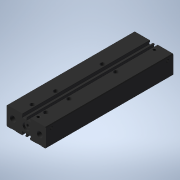
# Autodesk Inventor part: 529120 DFM---16-160-B-P-A-KF---(ZR) 150
Saved by Autodesk Inventor 2021 (Build 250183000, 183)
## iProperties
Created: 2025-06-19
Part Number: 529120 DFM---16-160-B-P-A-KF---(ZR) 150
Material: Generic
Catalog Web Link: www.cadenas.de
Description: DFM-B-(ZR)-Guide unit
Vendor: FESTO
Document SubType Name: Modeling
Designer: psAdmin
Manufacturer: FESTO
Mass: 360.15 g
Surface Area: 842.869 cm^2
Volume: 360.15 cm^3
Density: 1 g/cm^3
Appearance: PSOLRGB-175-175-175
Category: PARTsolutions
Company: FESTO
Title: 529120 DFM---16-160-B-P-A-KF---(ZR) 150
Author: Cadenas PARTsolutions
Comments: Guide unit
PSOL_IDENT_0: {$CADENAS_DATA/23d-libs/festo/parts/d/dfm/parts/dfm_b_z.prj},259 {VTYP=3D},{NB=529120 DFM---16-160-B
PSOL_IDENT_1: -P-A-KF---(ZR) 150},{LINA=529120 DFM---16-160-B-P-A-KF---(ZR) 150},{NN=DFM-B-(ZR)},{DATE=04.04.2025
PSOL_IDENT_2: 09:41:30},{GEOMDATE=04.04.2025 09:12:00},{VERSION=},{LINEID=550},{WBVAR=GEW,XHUB,CUSH,F,JUST},{WBNUM
PSOL_IDENT_3: ERIC=XHUB,CUSH,F,JUST}  {NB=529120 DFM---16-160-B-P-A-KF---(ZR) 150},{LINA=529120 DFM---16-160-B-P-A
PSOL_IDENT_4: -KF---(ZR) 150},{KT=1},{TNR=529120},{TYP=DFM},{GEW=-},{KDM=16},{D11=4.300},{XHUB=150},{HUB=160},{HUB
PSOL_IDENT_5: 1=[10:200]},{G=B},{CUSH=1},{F=2},{JUST=0},{VERS=1},{B1=67.000},{B2=65.000},{B3=45.000},{B4=4.500},{B
PSOL_IDENT_6: 5=58.000},{B6=22.000},{B7=23.000},{B8=23.500},{B9=20.000},{B10=10.500},{B11=46.000},{B12=9.500},{B13=
PSOL_IDENT_7: 46.000},{B14=21.300},{B15=24.400},{B16A=33.500},{B17A=0.000},{B18A=0.000},{B19A=0.000},{B20=0.000},{
PSOL_IDENT_8: B21=0.000},{D1=M 5},{D1P=5.000},{D1KDR=4.134},{D2=7.500},{D3=9.000},{D4=M 5},{D4P=5.000},{D4KDR=4.13
PSOL_IDENT_9: 4},{D5=5.000},{D6=4.3},{D6P=4.300},{D6KDR=3.242},{D7=10},{D7GF=12.000},{D7KF=10.000},{D8=5.000},{D9=
PSOL_IDENT_10: M 4},{D9P=4.000},{D9KDR=3.242},{D10=6.000},{FN=2},{FT=-KF},{E1=M 5},{EEMM=5.000},{EEKDR=4.134},{FE=
PSOL_IDENT_11: 0, '-', 1, 'AJ', 2, 'EJ', 3, 'AJ+EJ'},{H1=32.000},{H2=30.000},{H3=26.500},{H4=4.000},{H5=24.000},{H6=
PSOL_IDENT_12: 4.000},{H7=24.000},{H8=16.000},{H9=7.400},{H10=20.000},{H11=16.000},{H12A=16.000},{H13A=0.000},{H14A=
PSOL_IDENT_13: 16.000},{L1=264},{L2=58.000},{L3=10.000},{L4=12.000},{L5=9.800},{L6A=9.300},{L7=34},{L8=22.000},{L9=
PSOL_IDENT_14: 40},{L10=34.000},{L11=120},{L12=5.000},{L13A=4.000},{L14=0},{L15=0},{L16=0},{P1=0.000},{T1=12.000},{
PSOL_IDENT_15: T2=4.600},{T3=2.100},{T4=10.000},{T5=1.000},{T6=0.000},{T7=0.000},{T8=0.000},{T9=0.000},{SW1=10.000}
PSOL_IDENT_16: ,{SW2=10.000},{SW3=17.000},{SW4=0.000},{SW4D=0.000},{SW4KDR=0.000},{SW4M=0.000},{SW5=0.000},{SW6=0.0
PSOL_IDENT_17: 00},{SW7=0.000},{SW8=0.000},{SW9=0.000},{SW10=0.000},{SW2D=6.000},{SW2T=4.000},{ZZ=0},{MOD=1},{BR=0.
PSOL_IDENT_18: 000},{YB1=0.000},{YD1=0.000},{YD2=0.000},{YD3=0.000},{YD4=0.000},{YL1=0.000},{YL2=0.000},{YL3=0.000}
PSOL_IDENT_19: ,{YL4=0.000},{YL5=0.000},{YL6=0.000},{YL7=0.000},{YL14=0.000},{L14A=107.900},{L14Y=0.000},{L15A=0.00
PSOL_IDENT_20: 0},{L15Y=0.000},{L16A=107.900},{L16Y=0.000},{CUSHT=-P},{CUSHN=1},{JT=},{B16=0},{B17=0},{B18=0},{B19=
PSOL_IDENT_21: 0},{H12=0},{H13=0},{H14=0},{L6=0},{L13=0},{PPV1= 1, 'P', 2, 'PPV'},{PPV2= 1, 'P', 2, 'PPV'},{PPV= 1,
PSOL_IDENT_22: 'P', 2, 'PPV'},{JU= 0, '-', 1, 'AJ', 2, 'EJ', 3, 'AJ+EJ'},{FE1= 0, '-'},{VER=1.000},{RR=0.000},{VER
PSOL_IDENT_23: O=2},{A1=0.000},{A2=0.000},{A3=0.000},{A3D=0.000},{A4=0.000},{A5=0.000},{A6=0.000},{A7=0.000},{A8=0.
PSOL_IDENT_24: 000},{AD9=0.000},{A10=0.000},{A11=0.000},{A11D=0},{A12=0.000},{A13=0.000},{A14=0.000},{A15=0.000},{A
PSOL_IDENT_25: 16=0.000},{A17=0.000},{NPT=0},{BB=0.000},{LPPV=0.000},{DPPV=0.000},{LSLOT=8.000},{TSLOT=6.100},{YD33=
PSOL_IDENT_26: 0.000},{LD33=0.000}
NB: 529120 DFM---16-160-B-P-A-KF---(ZR) 150
NN: DFM-B-(ZR)
NT: Guide unit
NBSYN: $TNR. $TYP.-$GEW.-$KDM.-$HUB.-$G.$CUSHT.-A$FT.$JT.---(ZR) $XHUB.
LINA: 529120 DFM---16-160-B-P-A-KF---(ZR) 150
CATALOG: Festo
TNR: 529120
TYP: DFM
GEW: -
KDM: 16
D11: 4.3
XHUB: 150
HUB: 160
HUB1: [10:200]
G: B
CUSH: P
F: KF
JUST: -
B1: 67
B2: 65
B3: 45
B4: 4.5
B5: 58
B6: 22
B7: 23
B8: 23.5
B9: 20
B10: 10.5
B11: 46
B12: 9.5
B13: 46
B14: 21.3
B15: 24.4
B16A: 33.5
B17A: 0
B18A: 0
B19A: 0
B20: 0
B21: 0
D1: M 5
D1P: 5
D1KDR: 4.134
D2: 7.5
D3: 9
D4: M 5
D4P: 5
D4KDR: 4.134
D5: 5
D6: 4.3
D6P: 4.3
D6KDR: 3.242
D7GF: 12
D7KF: 10
D8: 5
D9: M 4
D9P: 4
D9KDR: 3.242
D10: 6
E1: M 5
EEKDR: 4.134
FE: 0, '-', 1, 'AJ', 2, 'EJ', 3, 'AJ+EJ'
H1: 32
H2: 30
H3: 26.5
H4: 4
H5: 24
H6: 4
H7: 24
H8: 16
H9: 7.4
H10: 20
H11: 16
H12A: 16
H13A: 0
H14A: 16
L1: 264
L2: 58
L3: 10
L4: 12
L5: 9.8
L6A: 9.3
L7: 34
L8: 22
L9: 40
L10: 34
L11: 120
L12: 5
L13A: 4
P1: 0
T1: 12
T2: 4.6
T3: 2.1
T4: 10
T5: 1
T6: 0
T7: 0
T8: 0
T9: 0
SW1: 10
SW2: 10
SW3: 17
SW4: 0
SW4D: 0
SW4KDR: 0
SW4M: 0
SW5: 0
SW6: 0
SW7: 0
SW8: 0
SW9: 0
SW10: 0
SW2D: 6
SW2T: 4
BR: 0
YB1: 0
YD1: 0
YD2: 0
YD3: 0
YD4: 0
YL1: 0
YL2: 0
YL3: 0
YL4: 0
YL5: 0
YL6: 0
YL7: 0
YL14: 0
L14A: 107.9
L14Y: 0
L15A: 0
L15Y: 0
L16A: 107.9
L16Y: 0
PPV1: 1, 'P', 2, 'PPV'
PPV2: 1, 'P', 2, 'PPV'
FE1: 0, '-'
VER: 1
RR: 0
A1: 0
A2: 0
A3: 0
A3D: 0
A4: 0
A5: 0
A6: 0
A7: 0
A8: 0
AD9: 0
A10: 0
A11: 0
A12: 0
A13: 0
A14: 0
A15: 0
A16: 0
A17: 0
BB: 0
LPPV: 0
DPPV: 0
LSLOT: 8
TSLOT: 6.1
YD33: 0
LD33: 0
SUPPLIER: FESTO
ARTICLENO: 529120 DFM---16-160-B-P-A-KF---(ZR) 150
BOMINFO: 529120 DFM---16-160-B-P-A-KF---(ZR) 150
CREATOR: CADENAS GmbH
Autodesk Inventor part; units mm, degrees
sketch "Sketch_1" plane through (0, 0, 0) normal (0, 0, 1) x (1, 0, 0)
  line L0 (-33.5, 15) -> (-33.5, -15)
  line L1 (-33.5, -15) -> (-32.5, -16)
  line L2 (-32.5, -16) -> (-26.3, -16)
  line L3 (-26.3, -16) -> (-26.0691, -15.6)
  arc A0 (-25.8959, -15.5) -> (-26.0691, -15.6) centre (-25.8959, -15.7) ccw
  line L4 (-25.8959, -15.5) -> (-18.1341, -15.5)
  arc A1 (-17.9609, -15.6) -> (-18.1341, -15.5) centre (-18.1341, -15.7) ccw
  line L5 (-17.9609, -15.6) -> (-17.73, -16)
  line L6 (-17.73, -16) -> (-7.1, -16)
  line L7 (-7.1, -16) -> (-6.6, -15.5)
  line L8 (-6.6, -15.5) -> (-6.6, -13.3)
  arc A2 (-6.6, -13.3) -> (-6.8, -13.1) centre (-6.8, -13.3) ccw
  line L9 (-6.8, -13.1) -> (-7.05, -13.1)
  arc A3 (-7.25, -12.9) -> (-7.05, -13.1) centre (-7.05, -12.9) ccw
  line L10 (-7.25, -12.9) -> (-7.25, -10.3)
  arc A4 (-6.85, -9.9) -> (-7.25, -10.3) centre (-6.85, -10.3) ccw
  line L11 (-6.85, -9.9) -> (-1.15, -9.9)
  arc A5 (-0.75, -10.3) -> (-1.15, -9.9) centre (-1.15, -10.3) ccw
  line L12 (-0.75, -10.3) -> (-0.75, -12.9)
  arc A6 (-0.95, -13.1) -> (-0.75, -12.9) centre (-0.95, -12.9) ccw
  line L13 (-0.95, -13.1) -> (-1.2, -13.1)
  arc A7 (-1.2, -13.1) -> (-1.4, -13.3) centre (-1.2, -13.3) ccw
  line L14 (-1.4, -13.3) -> (-1.4, -14.5)
  arc A8 (-1.4, -14.5) -> (-1, -14.9) centre (-1, -14.5) ccw
  line L15 (-1, -14.9) -> (1, -14.9)
  arc A9 (1, -14.9) -> (1.4, -14.5) centre (1, -14.5) ccw
  line L16 (1.4, -14.5) -> (1.4, -13.3)
  arc A10 (1.4, -13.3) -> (1.2, -13.1) centre (1.2, -13.3) ccw
  line L17 (1.2, -13.1) -> (0.95, -13.1)
  arc A11 (0.75, -12.9) -> (0.95, -13.1) centre (0.95, -12.9) ccw
  line L18 (0.75, -12.9) -> (0.75, -10.3)
  arc A12 (1.15, -9.9) -> (0.75, -10.3) centre (1.15, -10.3) ccw
  line L19 (1.15, -9.9) -> (6.85, -9.9)
  arc A13 (7.25, -10.3) -> (6.85, -9.9) centre (6.85, -10.3) ccw
  line L20 (7.25, -10.3) -> (7.25, -12.9)
  arc A14 (7.05, -13.1) -> (7.25, -12.9) centre (7.05, -12.9) ccw
  line L21 (7.05, -13.1) -> (6.8, -13.1)
  arc A15 (6.8, -13.1) -> (6.6, -13.3) centre (6.8, -13.3) ccw
  line L22 (6.6, -13.3) -> (6.6, -15.5)
  line L23 (6.6, -15.5) -> (7.1, -16)
  line L24 (7.1, -16) -> (17.73, -16)
  line L25 (17.73, -16) -> (17.9609, -15.6)
  arc A16 (18.1341, -15.5) -> (17.9609, -15.6) centre (18.1341, -15.7) ccw
  line L26 (18.1341, -15.5) -> (25.8959, -15.5)
  arc A17 (26.0691, -15.6) -> (25.8959, -15.5) centre (25.8959, -15.7) ccw
  line L27 (26.0691, -15.6) -> (26.3, -16)
  line L28 (26.3, -16) -> (32.5, -16)
  line L29 (32.5, -16) -> (33.5, -15)
  line L30 (33.5, -15) -> (33.5, 15)
  line L31 (33.5, 15) -> (32.5, 16)
  line L32 (32.5, 16) -> (7, 16)
  arc A18 (7, 16) -> (6.6, 15.6) centre (7, 15.6) ccw
  line L33 (6.6, 15.6) -> (6.6, 13.3)
  arc A19 (6.6, 13.3) -> (6.8, 13.1) centre (6.8, 13.3) ccw
  line L34 (6.8, 13.1) -> (7.05, 13.1)
  arc A20 (7.25, 12.9) -> (7.05, 13.1) centre (7.05, 12.9) ccw
  line L35 (7.25, 12.9) -> (7.25, 10.3)
  arc A21 (6.85, 9.9) -> (7.25, 10.3) centre (6.85, 10.3) ccw
  line L36 (6.85, 9.9) -> (1.15, 9.9)
  arc A22 (0.75, 10.3) -> (1.15, 9.9) centre (1.15, 10.3) ccw
  line L37 (0.75, 10.3) -> (0.75, 12.9)
  arc A23 (0.95, 13.1) -> (0.75, 12.9) centre (0.95, 12.9) ccw
  line L38 (0.95, 13.1) -> (1.2, 13.1)
  arc A24 (1.2, 13.1) -> (1.4, 13.3) centre (1.2, 13.3) ccw
  line L39 (1.4, 13.3) -> (1.4, 14.5)
  arc A25 (1.4, 14.5) -> (1, 14.9) centre (1, 14.5) ccw
  line L40 (1, 14.9) -> (-1, 14.9)
  arc A26 (-1, 14.9) -> (-1.4, 14.5) centre (-1, 14.5) ccw
  line L41 (-1.4, 14.5) -> (-1.4, 13.3)
  arc A27 (-1.4, 13.3) -> (-1.2, 13.1) centre (-1.2, 13.3) ccw
  line L42 (-1.2, 13.1) -> (-0.95, 13.1)
  arc A28 (-0.75, 12.9) -> (-0.95, 13.1) centre (-0.95, 12.9) ccw
  line L43 (-0.75, 12.9) -> (-0.75, 10.3)
  arc A29 (-1.15, 9.9) -> (-0.75, 10.3) centre (-1.15, 10.3) ccw
  line L44 (-1.15, 9.9) -> (-6.85, 9.9)
  arc A30 (-7.25, 10.3) -> (-6.85, 9.9) centre (-6.85, 10.3) ccw
  line L45 (-7.25, 10.3) -> (-7.25, 12.9)
  arc A31 (-7.05, 13.1) -> (-7.25, 12.9) centre (-7.05, 12.9) ccw
  line L46 (-7.05, 13.1) -> (-6.8, 13.1)
  arc A32 (-6.8, 13.1) -> (-6.6, 13.3) centre (-6.8, 13.3) ccw
  line L47 (-6.6, 13.3) -> (-6.6, 15.6)
  arc A33 (-6.6, 15.6) -> (-7, 16) centre (-7, 15.6) ccw
  line L48 (-7, 16) -> (-32.5, 16)
  line L49 (-32.5, 16) -> (-33.5, 15)
  constraints: 100 end point, 68 point on circle, 34 centre point
extrude "Extrusion1" add sketch "Sketch_1" against normal blind 218
sketch "Sketch2" plane through (7, 16, 0) normal (0, 1, 0) x (1, 0, 0)
  point P0 (4.5, 9.3)
hole "Hole1" at (11.5, 16, -9.3) direction (0, -1, 0) diameter 4.134 depth 5 countersink diameter 5 countersink angle 90 thread size "M5x0.8" class "6H" standard "ISO Metric profile"
sketch "Sketch3" plane through (7, 16, 0) normal (0, 1, 0) x (1, 0, 0)
  point P0 (4.5, 208.2)
hole "Hole2" at (11.5, 16, -208.2) direction (0, -1, 0) diameter 4.134 depth 5 countersink diameter 5 countersink angle 90 thread size "M5x0.8" class "6H" standard "ISO Metric profile"
sketch "Sketch4" plane through (33.5, -15, 0) normal (1, 0, 0) x (0, 0, -1)
  point P0 (9.3, 25.5)
hole "Hole3" at (33.5, 10.5, -9.3) direction (-1, 0, 0) diameter 4.134 depth 5 countersink diameter 5 countersink angle 90 thread size "M5x0.8" class "6H" standard "ISO Metric profile"
sketch "Sketch5" plane through (33.5, -15, 0) normal (1, 0, 0) x (0, 0, -1)
  point P0 (208.2, 25.5)
hole "Hole4" at (33.5, 10.5, -208.2) direction (-1, 0, 0) diameter 4.134 depth 5 countersink diameter 5 countersink angle 90 thread size "M5x0.8" class "6H" standard "ISO Metric profile"
sketch "Sketch_18" plane through (0, 0, -22) normal (0, 0, 1) x (1, 0, 0)
  line L0 (11.5, -16) -> (11.5, 16)
  line L1 (11.5, 16) -> (15.25, 16)
  line L2 (15.25, 16) -> (15.25, 11.4)
  line L3 (15.25, 11.4) -> (13.65, 11.4)
  line L4 (13.65, 11.4) -> (13.65, -4)
  line L5 (13.65, -4) -> (12.5, -4)
  line L6 (12.5, -4) -> (12.5, -13.9)
  line L7 (12.5, -13.9) -> (16, -13.9)
  line L8 (16, -13.9) -> (16, -16)
  line L9 (16, -16) -> (11.5, -16)
  line L10 (11.5, -16) -> (11.5, 16)
  constraints: 22 end point
revolve "Revolution1" cut sketch "Sketch_18" angle 360 about axis through (11.5, -16, -22) along (0, 1, 0)
sketch "Sketch_3" plane through (0, 0, -22) normal (0, 0, 1) x (1, 0, 0)
  line L0 (11.5, -13.9) -> (11.5, -4)
  line L1 (11.5, -4) -> (13.567, -4)
  line L2 (13.567, -4) -> (13.567, -13.467)
  line L3 (13.567, -13.467) -> (14, -13.9)
  line L4 (14, -13.9) -> (11.5, -13.9)
  line L5 (11.5, -13.9) -> (11.5, -4)
  constraints: 12 end point
revolve "Revolution2" cut sketch "Sketch_3" angle 360 about axis through (11.5, -13.9, -22) along (0, -1, 0)
thread "Thread1" size "M5x0.8" class "6H" standard "ISO Metric profile" full length
sketch "Sketch_19" plane through (0, 0, -22) normal (0, 0, 1) x (1, 0, 0)
  line L0 (-11.5, -16) -> (-11.5, 16)
  line L1 (-11.5, 16) -> (-7.75, 16)
  line L2 (-7.75, 16) -> (-7.75, 11.4)
  line L3 (-7.75, 11.4) -> (-9.35, 11.4)
  line L4 (-9.35, 11.4) -> (-9.35, -4)
  line L5 (-9.35, -4) -> (-10.5, -4)
  line L6 (-10.5, -4) -> (-10.5, -13.9)
  line L7 (-10.5, -13.9) -> (-7, -13.9)
  line L8 (-7, -13.9) -> (-7, -16)
  line L9 (-7, -16) -> (-11.5, -16)
  line L10 (-11.5, -16) -> (-11.5, 16)
  constraints: 22 end point
revolve "Revolution3" cut sketch "Sketch_19" angle 360 about axis through (-11.5, -16, -22) along (0, 1, 0)
sketch "Sketch_4" plane through (0, 0, -22) normal (0, 0, 1) x (1, 0, 0)
  line L0 (-11.5, -13.9) -> (-11.5, -4)
  line L1 (-11.5, -4) -> (-9.433, -4)
  line L2 (-9.433, -4) -> (-9.433, -13.467)
  line L3 (-9.433, -13.467) -> (-9, -13.9)
  line L4 (-9, -13.9) -> (-11.5, -13.9)
  line L5 (-11.5, -13.9) -> (-11.5, -4)
  constraints: 12 end point
revolve "Revolution4" cut sketch "Sketch_4" angle 360 about axis through (-11.5, -13.9, -22) along (0, -1, 0)
thread "Thread2" size "M5x0.8" class "6H" standard "ISO Metric profile" full length
sketch "Sketch_20" plane through (0, 0, -62) normal (0, 0, 1) x (1, 0, 0)
  line L0 (11.5, -16) -> (11.5, 16)
  line L1 (11.5, 16) -> (15.25, 16)
  line L2 (15.25, 16) -> (15.25, 11.4)
  line L3 (15.25, 11.4) -> (13.65, 11.4)
  line L4 (13.65, 11.4) -> (13.65, -4)
  line L5 (13.65, -4) -> (12.5, -4)
  line L6 (12.5, -4) -> (12.5, -16)
  line L7 (12.5, -16) -> (11.5, -16)
  line L8 (11.5, -16) -> (11.5, 16)
  constraints: 18 end point
revolve "Revolution5" cut sketch "Sketch_20" angle 360 about axis through (11.5, -16, -62) along (0, 1, 0)
sketch "Sketch_5" plane through (0, 0, -62) normal (0, 0, 1) x (1, 0, 0)
  line L0 (11.5, -16) -> (11.5, -4)
  line L1 (11.5, -4) -> (13.567, -4)
  line L2 (13.567, -4) -> (13.567, -15.567)
  line L3 (13.567, -15.567) -> (14, -16)
  line L4 (14, -16) -> (11.5, -16)
  line L5 (11.5, -16) -> (11.5, -4)
  constraints: 12 end point
revolve "Revolution6" cut sketch "Sketch_5" angle 360 about axis through (11.5, -16, -62) along (0, 1, 0)
thread "Thread3" size "M5x0.8" class "6H" standard "ISO Metric profile" full length
sketch "Sketch_21" plane through (0, 0, -62) normal (0, 0, 1) x (1, 0, 0)
  line L0 (-11.5, -16) -> (-11.5, 16)
  line L1 (-11.5, 16) -> (-7.75, 16)
  line L2 (-7.75, 16) -> (-7.75, 11.4)
  line L3 (-7.75, 11.4) -> (-9.35, 11.4)
  line L4 (-9.35, 11.4) -> (-9.35, -4)
  line L5 (-9.35, -4) -> (-10.5, -4)
  line L6 (-10.5, -4) -> (-10.5, -16)
  line L7 (-10.5, -16) -> (-11.5, -16)
  line L8 (-11.5, -16) -> (-11.5, 16)
  constraints: 18 end point
revolve "Revolution7" cut sketch "Sketch_21" angle 360 about axis through (-11.5, -16, -62) along (0, 1, 0)
sketch "Sketch_6" plane through (0, 0, -62) normal (0, 0, 1) x (1, 0, 0)
  line L0 (-11.5, -16) -> (-11.5, -4)
  line L1 (-11.5, -4) -> (-9.433, -4)
  line L2 (-9.433, -4) -> (-9.433, -15.567)
  line L3 (-9.433, -15.567) -> (-9, -16)
  line L4 (-9, -16) -> (-11.5, -16)
  line L5 (-11.5, -16) -> (-11.5, -4)
  constraints: 12 end point
revolve "Revolution8" cut sketch "Sketch_6" angle 360 about axis through (-11.5, -16, -62) along (0, 1, 0)
thread "Thread4" size "M5x0.8" class "6H" standard "ISO Metric profile" full length
sketch "Sketch_22" plane through (0, 0, -142) normal (0, 0, 1) x (1, 0, 0)
  line L0 (11.5, -16) -> (11.5, 16)
  line L1 (11.5, 16) -> (15.25, 16)
  line L2 (15.25, 16) -> (15.25, 11.4)
  line L3 (15.25, 11.4) -> (13.65, 11.4)
  line L4 (13.65, 11.4) -> (13.65, -4)
  line L5 (13.65, -4) -> (12.5, -4)
  line L6 (12.5, -4) -> (12.5, -16)
  line L7 (12.5, -16) -> (11.5, -16)
  line L8 (11.5, -16) -> (11.5, 16)
  constraints: 18 end point
revolve "Revolution9" cut sketch "Sketch_22" angle 360 about axis through (11.5, -16, -142) along (0, 1, 0)
sketch "Sketch_8" plane through (0, 0, -142) normal (0, 0, 1) x (1, 0, 0)
  line L0 (11.5, -16) -> (11.5, -4)
  line L1 (11.5, -4) -> (13.567, -4)
  line L2 (13.567, -4) -> (13.567, -15.567)
  line L3 (13.567, -15.567) -> (14, -16)
  line L4 (14, -16) -> (11.5, -16)
  line L5 (11.5, -16) -> (11.5, -4)
  constraints: 12 end point
revolve "Revolution10" cut sketch "Sketch_8" angle 360 about axis through (11.5, -16, -142) along (0, 1, 0)
thread "Thread5" size "M5x0.8" class "6H" standard "ISO Metric profile" full length
sketch "Sketch_23" plane through (0, 0, -142) normal (0, 0, 1) x (1, 0, 0)
  line L0 (-11.5, -16) -> (-11.5, 16)
  line L1 (-11.5, 16) -> (-7.75, 16)
  line L2 (-7.75, 16) -> (-7.75, 11.4)
  line L3 (-7.75, 11.4) -> (-9.35, 11.4)
  line L4 (-9.35, 11.4) -> (-9.35, -4)
  line L5 (-9.35, -4) -> (-10.5, -4)
  line L6 (-10.5, -4) -> (-10.5, -16)
  line L7 (-10.5, -16) -> (-11.5, -16)
  line L8 (-11.5, -16) -> (-11.5, 16)
  constraints: 18 end point
revolve "Revolution11" cut sketch "Sketch_23" angle 360 about axis through (-11.5, -16, -142) along (0, 1, 0)
sketch "Sketch_7" plane through (0, 0, -142) normal (0, 0, 1) x (1, 0, 0)
  line L0 (-11.5, -16) -> (-11.5, -4)
  line L1 (-11.5, -4) -> (-9.433, -4)
  line L2 (-9.433, -4) -> (-9.433, -15.567)
  line L3 (-9.433, -15.567) -> (-9, -16)
  line L4 (-9, -16) -> (-11.5, -16)
  line L5 (-11.5, -16) -> (-11.5, -4)
  constraints: 12 end point
revolve "Revolution12" cut sketch "Sketch_7" angle 360 about axis through (-11.5, -16, -142) along (0, 1, 0)
thread "Thread6" size "M5x0.8" class "6H" standard "ISO Metric profile" full length
sketch "Sketch18" plane through (-33.5, -15, 0) normal (-1, 0, 0) x (0, 0, 1)
  point P0 (-22, 3)
hole "Hole5" at (-33.5, -12, -22) direction (1, 0, 0) diameter 4.134 depth 12.14 tip angle 120 countersink diameter 5 countersink angle 90 thread size "M5x0.8" class "6H" standard "ISO Metric profile"
sketch "Sketch19" plane through (-33.5, -15, 0) normal (-1, 0, 0) x (0, 0, 1)
  point P0 (-22, 27)
hole "Hole6" at (-33.5, 12, -22) direction (1, 0, 0) diameter 4.134 depth 12.14 tip angle 120 countersink diameter 5 countersink angle 90 thread size "M5x0.8" class "6H" standard "ISO Metric profile"
sketch "Sketch20" plane through (-33.5, -15, 0) normal (-1, 0, 0) x (0, 0, 1)
  point P0 (-62, 3)
hole "Hole7" at (-33.5, -12, -62) direction (1, 0, 0) diameter 4.134 depth 12.14 tip angle 120 countersink diameter 5 countersink angle 90 thread size "M5x0.8" class "6H" standard "ISO Metric profile"
sketch "Sketch21" plane through (-33.5, -15, 0) normal (-1, 0, 0) x (0, 0, 1)
  point P0 (-62, 27)
hole "Hole8" at (-33.5, 12, -62) direction (1, 0, 0) diameter 4.134 depth 12.14 tip angle 120 countersink diameter 5 countersink angle 90 thread size "M5x0.8" class "6H" standard "ISO Metric profile"
sketch "Sketch22" plane through (-33.5, -15, 0) normal (-1, 0, 0) x (0, 0, 1)
  point P0 (-142, 3)
hole "Hole9" at (-33.5, -12, -142) direction (1, 0, 0) diameter 4.134 depth 12.14 tip angle 120 countersink diameter 5 countersink angle 90 thread size "M5x0.8" class "6H" standard "ISO Metric profile"
sketch "Sketch23" plane through (-33.5, -15, 0) normal (-1, 0, 0) x (0, 0, 1)
  point P0 (-142, 27)
hole "Hole10" at (-33.5, 12, -142) direction (1, 0, 0) diameter 4.134 depth 12.14 tip angle 120 countersink diameter 5 countersink angle 90 thread size "M5x0.8" class "6H" standard "ISO Metric profile"
sketch "Sketch24" plane through (0, 0, -218) normal (0, 0, -1) x (-1, 0, 0)
  point P0 (29, -12)
hole "Hole11" at (-29, -12, -218) direction (0, 0, 1) diameter 4.134 depth 12.14 tip angle 120 countersink diameter 5 countersink angle 90 thread size "M5x0.8" class "6H" standard "ISO Metric profile"
sketch "Sketch25" plane through (0, 0, -218) normal (0, 0, -1) x (-1, 0, 0)
  point P0 (29, 12)
hole "Hole12" at (-29, 12, -218) direction (0, 0, 1) diameter 4.134 depth 12.14 tip angle 120 countersink diameter 5 countersink angle 90 thread size "M5x0.8" class "6H" standard "ISO Metric profile"
sketch "Sketch26" plane through (0, 0, -218) normal (0, 0, -1) x (-1, 0, 0)
  point P0 (-29, -12)
hole "Hole13" at (29, -12, -218) direction (0, 0, 1) diameter 4.134 depth 12.14 tip angle 120 countersink diameter 5 countersink angle 90 thread size "M5x0.8" class "6H" standard "ISO Metric profile"
sketch "Sketch27" plane through (0, 0, -218) normal (0, 0, -1) x (-1, 0, 0)
  point P0 (12.2, 0)
hole "Hole14" at (-12.2, 0, -218) direction (0, 0, 1) diameter 5 depth 1
sketch "Sketch28" plane through (0, 0, -218) normal (0, 0, -1) x (-1, 0, 0)
  point P0 (-12.2, 0)
hole "Hole15" at (12.2, 0, -218) direction (0, 0, 1) diameter 5 depth 1
sketch "Skizze_1" plane through (0, 0, 0) normal (1, 0, 0) x (0, 1, 0)
  line L0 (0, -171.95) -> (0, 0)
  line L1 (0, 0) -> (6.25, 0)
  line L2 (6.25, 0) -> (6.25, -3.2)
  line L3 (6.25, -3.2) -> (3, -3.2)
  line L4 (3, -3.2) -> (3, -13.95)
  line L5 (3, -13.95) -> (8, -13.95)
  line L6 (8, -13.95) -> (8, -171.95)
  line L7 (8, -171.95) -> (0, -171.95)
  line L8 (0, -171.95) -> (0, 0)
  constraints: 18 end point
revolve "Revolution13" cut sketch "Skizze_1" angle 360 about axis through (0, 0, -171.95) along (0, 0, 1)
sketch "Skizze_5" plane through (0, 0, -22) normal (0, 0, 1) x (1, 0, 0)
  line L0 (-32.5, 0) -> (-33.5, 0)
  line L1 (-33.5, 0) -> (-33.5, 2.5)
  line L2 (-33.5, 2.5) -> (-32.5, 2.5)
  line L3 (-32.5, 2.5) -> (-32.5, 0)
  line L4 (-32.5, 0) -> (-33.5, 0)
  constraints: 10 end point
revolve "Revolution14" cut sketch "Skizze_5" angle 360 about axis through (-32.5, 0, -22) along (1, 0, 0)
sketch "Skizze_6" plane through (0, 0, -62) normal (0, 0, 1) x (1, 0, 0)
  line L0 (-32.5, 0) -> (-33.5, 0)
  line L1 (-33.5, 0) -> (-33.5, 2.5)
  line L2 (-33.5, 2.5) -> (-32.5, 2.5)
  line L3 (-32.5, 2.5) -> (-32.5, 0)
  line L4 (-32.5, 0) -> (-33.5, 0)
  constraints: 10 end point
revolve "Revolution15" cut sketch "Skizze_6" angle 360 about axis through (-32.5, 0, -62) along (1, 0, 0)
sketch "Sketch32" plane through (0, 0, 0) normal (0, 0, 1) x (1, 0, 0)
  point P0 (-23, 0)
hole "Hole16" at (-23, 0, 0) direction (0, 0, -1) diameter 10 depth 218
sketch "Sketch33" plane through (0, 0, 0) normal (0, 0, 1) x (1, 0, 0)
  point P0 (23, 0)
hole "Hole17" at (23, 0, 0) direction (0, 0, -1) diameter 10 depth 218
ref_plane "DIM_EE_1_TOP_XY" through (11.5, 16, -9.3) normal (0, -1, 0) x (1, 0, 0)
ref_plane "DIM_EE_1_TOP_YZ" through (11.5, 16, -9.3) normal (1, 0, 0) x (0, 0, 1)
ref_plane "DIM_EE_1_TOP_ZX" through (11.5, 16, -9.3) normal (0, 0, 1) x (0, -1, 0)
ref_plane "HUELSE1_1_XY" through (-32.5, 0, -22) normal (1, 0, 0) x (0, 0, -1)
ref_plane "HUELSE1_1_YZ" through (-32.5, 0, -22) normal (0, 0, -1) x (0, 1, 0)
ref_plane "HUELSE1_1_ZX" through (-32.5, 0, -22) normal (0, 1, 0) x (1, 0, 0)
ref_plane "HUELSE1_2_XY" through (-32.5, 0, -62) normal (1, 0, 0) x (0, 0, -1)
ref_plane "HUELSE1_2_YZ" through (-32.5, 0, -62) normal (0, 0, -1) x (0, 1, 0)
ref_plane "HUELSE1_2_ZX" through (-32.5, 0, -62) normal (0, 1, 0) x (1, 0, 0)
ref_plane "HUELSE2_1_XY" through (11.5, -13.9, -22) normal (0, 1, 0) x (1, 0, 0)
ref_plane "HUELSE2_1_YZ" through (11.5, -13.9, -22) normal (1, 0, 0) x (0, 0, -1)
ref_plane "HUELSE2_1_ZX" through (11.5, -13.9, -22) normal (0, 0, -1) x (0, 1, 0)
ref_plane "HUELSE2_2_XY" through (-11.5, -13.9, -22) normal (0, 1, 0) x (1, 0, 0)
ref_plane "HUELSE2_2_YZ" through (-11.5, -13.9, -22) normal (1, 0, 0) x (0, 0, -1)
ref_plane "HUELSE2_2_ZX" through (-11.5, -13.9, -22) normal (0, 0, -1) x (0, 1, 0)
ref_plane "PIN_1_XY" through (11.5, 16, -9.3) normal (0, 1, 0) x (1, 0, 0)
ref_plane "PIN_1_YZ" through (11.5, 16, -9.3) normal (1, 0, 0) x (0, 0, -1)
ref_plane "PIN_1_ZX" through (11.5, 16, -9.3) normal (0, 0, -1) x (0, 1, 0)
ref_plane "PIN_2_XY" through (11.5, 16, -208.2) normal (0, 1, 0) x (1, 0, 0)
ref_plane "PIN_2_YZ" through (11.5, 16, -208.2) normal (1, 0, 0) x (0, 0, -1)
ref_plane "PIN_2_ZX" through (11.5, 16, -208.2) normal (0, 0, -1) x (0, 1, 0)
ref_plane "SENSOR1_XY" through (4, 9.9, -35) normal (0, 0, 1) x (1, 0, 0)
ref_plane "SENSOR1_YZ" through (4, 9.9, -35) normal (1, 0, 0) x (0, 1, 0)
ref_plane "SENSOR1_ZX" through (4, 9.9, -35) normal (0, 1, 0) x (0, 0, 1)
ref_plane "SENSOR2_XY" through (-4, 12, -173) normal (0, 0, 1) x (1, 0, 0)
ref_plane "SENSOR2_YZ" through (-4, 12, -173) normal (1, 0, 0) x (0, 1, 0)
ref_plane "SENSOR2_ZX" through (-4, 12, -173) normal (0, 1, 0) x (0, 0, 1)
ref_plane "SLOT_XY" through (4, 26, 0) normal (0, 0, 1) x (1, 0, 0)
ref_plane "SLOT_YZ" through (4, 26, 0) normal (1, 0, 0) x (0, 1, 0)
ref_plane "SLOT_ZX" through (4, 26, 0) normal (0, 1, 0) x (0, 0, 1)
ref_plane "TO_DUMMY_XY" through (0, 0, 0) normal (0, 1, 0) x (1, 0, 0)
ref_plane "TO_DUMMY_YZ" through (0, 0, 0) normal (1, 0, 0) x (0, 0, -1)
ref_plane "TO_DUMMY_ZX" through (0, 0, 0) normal (0, 0, -1) x (0, 1, 0)
ref_plane "zylinder_dfm_XY" through (0, 0, 0) normal (0, 0, 1) x (1, 0, 0)
ref_plane "zylinder_dfm_YZ" through (0, 0, 0) normal (1, 0, 0) x (0, 1, 0)
ref_plane "zylinder_dfm_ZX" through (0, 0, 0) normal (0, 1, 0) x (0, 0, 1)
body "Solid1"
